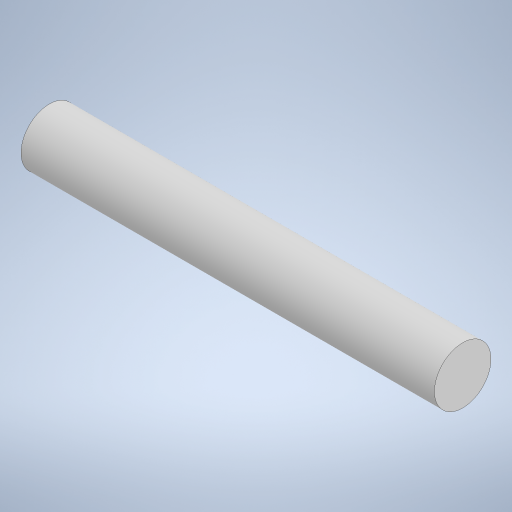
# Autodesk Inventor part: Enclosure_Lightsaber
Saved by Autodesk Inventor 2023 (Build 270158030, 158C)
## iProperties
Created: 2024-02-03
Part Number: Enclosure_Lightsaber
Material: Generic
Document SubType Name: Modeling
Designer: Fabian
Density: 1 g/cm^3
Appearance: Default
Author: Fabian
Autodesk Inventor part; units mm, degrees
ref_plane "YZ Plane" through (0, 0, 0) normal (1, 0, 0) x (0, 1, 0)
ref_plane "XZ Plane" through (0, 0, 0) normal (0, 1, 0) x (-1, 0, 0)
ref_plane "XY Plane" through (0, 0, 0) normal (0, 0, 1) x (1, 0, 0)
sketch "Sketch1" plane through (0, 0, 0) normal (1, 0, 0) x (0, 1, 0)
  circle A0 centre (0, 0) radius 0.95
  dimension "d0" = 1.9
  constraints: 1 centre point, 1 coincident
  measures "d0" diameter of A0
extrude "Extrusion1" add sketch "Sketch1" along normal blind 13.9
body "Solid1"
